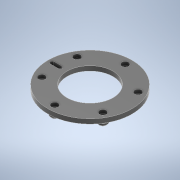
# Autodesk Inventor part: top
Saved by Autodesk Inventor 2022 (Build 260153000, 153)
## iProperties
Created: 2022-02-18
Part Number: top
Material: Genérico
Document SubType Name: Modeling
Designer: JK
Density: 1 g/cm^3
Appearance: Suave - Negro
Author: JK
Autodesk Inventor part; units mm, degrees
ref_plane "YZ Plane" through (0, 0, 0) normal (1, 0, 0) x (0, 1, 0)
ref_plane "XZ Plane" through (0, 0, 0) normal (0, 1, 0) x (-1, 0, 0)
ref_plane "XY Plane" through (0, 0, 0) normal (0, 0, 1) x (1, 0, 0)
sketch "Boceto1" plane through (0, 0, 0) normal (0, 1, 0) x (-1, 0, 0)
  circle A0 centre (0, 0) radius 36.5
  circle A1 centre (0, 0) radius 20
  dimension "d0" = 73
  dimension "d1" = 40
  constraints: 2 centre point, 2 coincident
  measures "d0" diameter of A0
  measures "d1" diameter of A1
extrude "Extrusión1" add sketch "Boceto1" along normal blind 4
sketch "Boceto2" plane through (0, 0, 0) normal (0, -1, 0) x (1, 0, 0)
  circle A0 centre (0, 30.6) radius 3.75
  point P0 (0, 0)
  dimension "d4" = 7.5
  dimension "d5" = 30.6
  constraints: 1 centre point
  measures "d4" diameter of A0
  measures "d5" distance of A0.centre point (0, 0)
extrude "Extrusión2" add sketch "Boceto2" along normal blind 3.3
sketch "Boceto3" plane through (0, -3.3, 30.6) normal (0, -1, 0) x (1, 0, 0)
  circle A0 centre (0, 0) radius 1.6
  point P0 (0, -30.6)
  dimension "d8" = 3.2
  constraints: 1 centre point
  measures "d8" diameter of A0
extrude "Extrusión3" cut sketch "Boceto3" against normal through all
fillet "Empalme1" radius 2 1 edges at (-3.75, 0, 30.6)
pattern_circular "Patrón circular1" count 6 over 360 about axis through (0, 0, 0) along (0, 1, 0) of "Extrusión2", "Extrusión3", "Empalme1"
sketch "Boceto4" plane through (0, 4, 0) normal (0, 1, 0) x (1, 0, 0)
  circle A0 centre (-26, 0) radius 1.65
  circle A1 centre (-33, 0) radius 1.65
  line L0 (-26, 1.65) -> (-33, 1.65)
  line L1 (-33, 1.65) -> (-33, -1.65)
  line L2 (-33, -1.65) -> (-26, -1.65)
  line L3 (-26, -1.65) -> (-26, 1.65)
  point P0 (0, 0)
  dimension "d14" = 3.3
  dimension "d15" = 26
  dimension "d16" = 7
  constraints: 8 end point, 5 horizontal, 2 parallel, 1 horizontal alignment, 1 midpoint, 1 perpendicular, 6 other
  measures "d15" distance from line of point (0, 0) L3
  measures "d16" distance of L1.end L2.end
extrude "Extrusión4" cut sketch "Boceto4" against normal through all
sketch "Boceto5" plane through (26.5004, -3.3, 15.3) normal (0, -1, 0) x (1, 0, 0)
  circle A0 centre (-53.0008, 0) radius 1.6 projected
  circle A1 centre (-53.0008, 0) radius 2.95
  point P0 (-26.5004, -15.3)
  dimension "d20" = 5.9
  constraints: 1 centre point, 1 coincident
  measures "d20" diameter of A1
extrude "Extrusión5" add sketch "Boceto5" along normal blind 1
pattern_circular "Patrón circular2" count 6 over 360 about axis through (0, 0, 0) along (0, 1, 0) of "Extrusión5"
sketch "Boceto6" plane through (0, 4, 0) normal (0, 1, 0) x (1, 0, 0)
  circle A0 centre (-26.5004, -15.3) radius 1.6 projected
  circle A1 centre (-26.5004, -15.3) radius 3
  point P0 (0, 0)
  dimension "d29" = 6
  constraints: 1 centre point, 1 coincident
  measures "d29" diameter of A1
extrude "Extrusión6" cut sketch "Boceto6" against normal blind 3
chamfer "Chaflán2" distance 1.4 angle 45 1 edges at (-27.3004, 1, 13.9144)
pattern_circular "Patrón circular3" count 6 over 360 about axis through (0, 0, 0) along (0, 1, 0) of "Extrusión6"
chamfer "Chaflán3" distance 1.4 angle 45 5 edges at (-25.7004, 1, -16.6856) (1.6, 1, -30.6) (27.3004, 1, -13.9144) (25.7004, 1, 16.6856) (-1.6, 1, 30.6)
